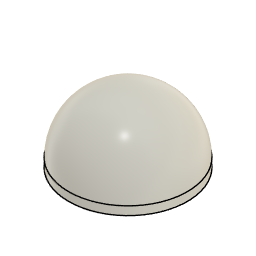
Bille v2 (Autodesk Fusion 360 design; units mm, degrees)
Autodesk Fusion 360 part; units mm, degrees
sketch "Esquisse1" plane through (0, 0, 0) normal (0, 0, 1) x (1, 0, 0)
  circle A0 centre (0, 0) radius 7
  line L0 (0, 0) -> (0, 7)
  line L1 (0, 0) -> (0, -7)
  dimension "d1" = 14
  constraint coincident A0.centre L0.start
  constraint coincident A0 L0.end
  constraint vertical L0
  constraint coincident A0 L1.end
  constraint parallel L0 L1
  measures "d1" diameter of A0
revolve "Révolution1" add sketch "Esquisse1" angle 180 about axis through (0, 0, 0) along (0, 1, 0) contours A0 L0 L1 picked at (-0.3478, -4.6406)
extrude "Extrusion1" add 2 faces at (-0.3478, -4.6406, 0) (0.3478, -4.6406, 0) along direction (0, 0, -1) blind 1
